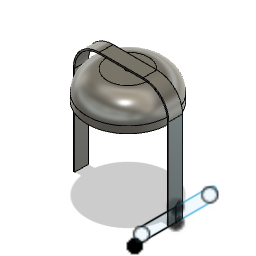
test_6 v2 (Autodesk Fusion 360 design; units mm, degrees)
Autodesk Fusion 360 part; units mm, degrees
sketch "Sketch1" plane through (0, 0, 0) normal (0, 0, 1) x (1, 0, 0)
  line L0 (0, 0) -> (150, 0)
  line L1 (150, 0) -> (150, 25)
  line L2 (75, 100) -> (0, 100)
  line L3 (0, 100) -> (0, 0)
  arc A0 (150, 25) -> (75, 100) centre (75, 25) ccw
  dimension "d1" = 150
  dimension "d2" = 100
  dimension "d3" = 75
  constraint horizontal L0
  constraint vertical L1
  constraint horizontal L2
  constraint vertical L3
  constraint coincident L0.start L3.end
  constraint tangent L1 A0
  constraint tangent L2 A0
  measures "d1" distance of L0.start L0.end
  measures "d2" distance of L0.start L2.end
  measures "d3" radius of A0
revolve "Revolve1" add sketch "Sketch1" angle 360 about axis through (0, 100, 0) along (0, -1, 0) makes body 1
sketch "Sketch2" plane through (0, 0, 0) normal (0, 0, 1) x (1, 0, 0)
  line L0 (0, 100) -> (-10, 100)
  line L1 (-10, 100) -> (-10, 120)
  line L2 (-10, 120) -> (0, 120)
  line L3 (0, 120) -> (0, 100)
  constraint horizontal L0
  constraint vertical L1
  constraint horizontal L2
  constraint vertical L3
revolve "Revolve2" add sketch "Sketch2" angle 360 about axis through (0, 120, 0) along (0, -1, 0) bodies 1
sketch "Sketch3" plane through (0, 0, 0) normal (0, 0, 1) x (1, 0, 0)
  line L0 (-0.1829, 119.7073) -> (-80, 119.7073)
  arc A0 (-80, 119.7073) -> (-170, 29.7073) centre (-80, 29.7073) ccw
  line L1 (-170, 29.7073) -> (-170, -0.2927)
  line L2 (-170, -0.2927) -> (-170, -300.2927)
  line L3 (0, 119.7073) -> (-80, 119.7073)
  arc A1 (-80, 119.7073) -> (-170, 29.7073) centre (-80, 29.7073) ccw
  line L4 (-170, -0.2927) -> (-170, -300.2927)
  line L5 (-170, 29.7073) -> (-170, -0.2927)
  line L6 (0, 119.7073) -> (80, 119.7073)
  arc A2 (170, 29.7073) -> (80, 119.7073) centre (80, 29.7073) ccw
  line L7 (170, 29.7073) -> (170, -0.2927)
  line L8 (170, -0.2927) -> (170, -300.2927)
  line L9 (170, -300.2927) -> (175, -300.2927)
  line L10 (175, -300.2927) -> (175, 31.7247)
  line L11 (0, 125) -> (80, 125)
  line L12 (80, 125) -> (81.0467, 125)
  arc A3 (175, 31.7247) -> (81.0467, 125) centre (81.0467, 31.0442) ccw
  line L13 (0, 125) -> (-80, 125)
  arc A4 (-80, 125) -> (-175, 32.0149) centre (-81.0006, 31.0004) ccw
  line L14 (-175, -300.2927) -> (-175, 32.0149)
  line L15 (-170, -300.2927) -> (-175, -300.2927)
  dimension "d6" = 300
  dimension "d7" = 300
  dimension "d8" = 5
  constraint horizontal L0
  constraint tangent L0 A0
  constraint tangent A0 L1
  constraint perpendicular L0 L1
  constraint perpendicular L0 L2
  constraint horizontal L3
  constraint tangent L3 A1
  constraint tangent A1 L5
  constraint perpendicular L3 L5
  constraint perpendicular L3 L4
  constraint perpendicular L8 L9
  constraint vertical L10
  constraint tangent L12 A3
  measures "d6" distance of L1.end L2.end
  measures "d7" distance of L2.end L1.end
  measures "d8" distance of L8.end L9.end
extrude "Extrude1" add sketch "Sketch3" along normal blind 25 and the other way blind 25 separate body makes body 2
sketch "Sketch4" plane through (175, 0, 0) normal (1, 0, 0) x (0, 0, -1)
  line L0 (25, 31.7247) -> (-25, 31.7247)
  line L1 (-25, 31.7247) -> (-25, -300.2927)
  line L2 (-25, -300.2927) -> (25, -300.2927)
  line L3 (25, -300.2927) -> (25, 31.7247)
  line L4 (0, -300.2927) -> (-125, -300.2927)
  line L5 (-125, -250.2927) -> (0, -250.2927)
  line L6 (0, -250.2927) -> (0, -300.2927)
  line L7 (125, -250.2927) -> (0, -250.2927)
  line L8 (0, -300.2927) -> (125, -300.2927)
  arc A0 (-125, -250.2927) -> (-150, -275.2927) centre (-125, -275.2927) ccw
  arc A1 (-150, -275.2927) -> (-125, -300.2927) centre (-125, -275.2927) ccw
  arc A2 (150, -275.2927) -> (125, -250.2927) centre (125, -275.2927) ccw
  arc A3 (125, -300.2927) -> (150, -275.2927) centre (125, -275.2927) ccw
  point P0 (-150, -300.2927)
  dimension "d13" = 150
  dimension "d14" = 50
  dimension "d15" = 25
  constraint horizontal L4
  constraint horizontal L5
  constraint vertical L6
  constraint midpoint L2 L4.start
  constraint symmetric L4.start L6 L8.start
  constraint symmetric L5.end L6 L7.end
  constraint tangent L5 A0
  constraint coincident P0 L4
  constraint tangent L4 A1
  constraint equal A0 A1
  constraint coincident A0.end A1.start
  constraint tangent L7 A2
  constraint equal A0 A2
  constraint tangent L8 A3
  constraint equal A0 A3
  constraint coincident A2.start A3.end
  measures "d13" distance of L4.start P0
  measures "d14" distance of L4.start L5.end
  measures "d15" radius of A0
